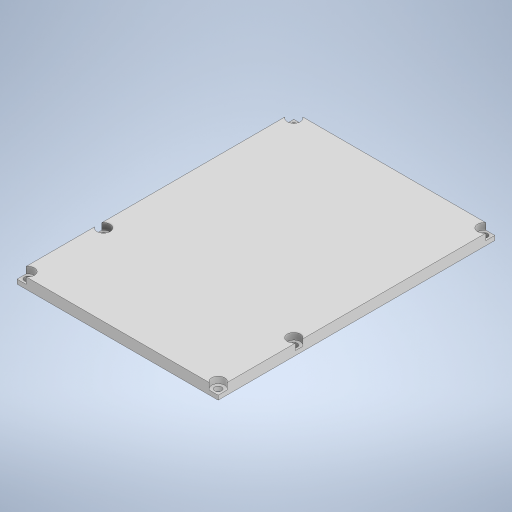
# Autodesk Inventor part: 싸피 뚜껑 원본
Saved by Autodesk Inventor 2023 (Build 270158000, 158)
## iProperties
Created: 2023-08-15
Part Number: 싸피 뚜껑 원본
Material: 일반
Document SubType Name: Sheet Metal
Designer: jin
Density: 1 g/cm^3
Sheet Metal Rule: 기본값_mm
Appearance: 기본값
Author: jin
## iProperties of the stored document 싸피 뚜껑_3D 인쇄.ipt
Created: 2023-08-16
Part Number: 싸피 뚜껑_3D 인쇄
Material: 일반
Document SubType Name: Modeling
Designer: jin
Density: 1 g/cm^3
Appearance: 기본값
Author: jin
Autodesk Inventor part; units mm, degrees
ref_plane "YZ Plane" through (0, 0, 0) normal (1, 0, 0) x (0, 1, 0)
ref_plane "XZ Plane" through (0, 0, 0) normal (0, 1, 0) x (-1, 0, 0)
ref_plane "XY Plane" through (0, 0, 0) normal (0, 0, 1) x (1, 0, 0)
sketch "스케치1" plane through (0, 0, 0) normal (0, 1, 0) x (-1, 0, 0)
  line L0 (0, 0) -> (93, 0)
  line L1 (93, 0) -> (93, -128)
  line L2 (93, -128) -> (0, -128)
  line L3 (0, -128) -> (0, 0)
  dimension "d0" = 93
  dimension "d1" = 128
  constraints: 8 end point, 2 parallel, 1 horizontal, 1 perpendicular
  measures "d0" distance of L1.end L2.end
  measures "d1" distance of L0.end L1.end
extrude "돌출1" add sketch "스케치1" along normal blind 5
sketch "스케치2" plane through (0, 5, 0) normal (0, 1, 0) x (1, 0, 0)
  line L0 (-93, 0) -> (0, 0) projected
  line L1 (0, 0) -> (0, 5)
  line L2 (0, 0) -> (0, 128) projected
  line L3 (0, 5) -> (0, 35)
  line L4 (0, 35) -> (0, 40)
  line L5 (0, 5) -> (-93, 5)
  line L6 (-93, 128) -> (-93, 0) projected
  line L7 (-93, 0) -> (-88, 0)
  line L8 (-88, 0) -> (-88, 5)
  line L9 (-88, 5) -> (-88, 35)
  line L10 (-88, 35) -> (0, 35)
  line L11 (-88, 35) -> (-93, 35)
  line L12 (-93, 35) -> (-93, 40)
  line L13 (-93, 40) -> (0, 40)
  line L14 (-88, 35) -> (-88, 40)
  line L15 (-88, 40) -> (-88, 128)
  line L16 (0, 128) -> (-93, 128) projected
  line L17 (-88, 128) -> (-88, 123)
  line L18 (-93, 123) -> (-88, 123)
  line L19 (-88, 123) -> (0, 123)
  line L20 (0, 128) -> (0, 125.5)
  line L21 (0, 125.5) -> (-2.5, 125.5)
  line L22 (-93, 128) -> (-93, 125.5)
  line L23 (-93, 125.5) -> (-90.5, 125.5)
  line L24 (-93, 40) -> (-93, 37.5)
  line L25 (-93, 37.5) -> (-90.5, 37.5)
  line L26 (0, 40) -> (0, 37.5)
  line L27 (0, 37.5) -> (-2.5, 37.5)
  line L28 (-93, 0) -> (-93, 2.5)
  line L29 (-93, 2.5) -> (-90.5, 2.5)
  line L30 (0, 0) -> (0, 2.5)
  line L31 (0, 5) -> (0, 2.5)
  line L32 (0, 2.5) -> (-2.5, 2.5)
  dimension "d4" = 5
  dimension "d5" = 30
  dimension "d6" = 5
  dimension "d7" = 5
  dimension "d8" = 30
  dimension "d9" = 5
  dimension "d10" = 5
  dimension "d11" = 2.5
  constraints: 58 end point, 20 point on line, 7 horizontal, 4 perpendicular, 2 midpoint, 1 collinear
  measures "d4" distance of L0.end L1.end
  measures "d5" distance of L1.end L3.end
  measures "d6" distance of L3.end L4.end
  measures "d7" distance of L0.start L7.end
  measures "d8" distance of L8.end L9.end
  measures "d9" distance of L11.end L12.end
  measures "d10" distance of L15.end L17.end
  measures "d11" distance of L20.end L21.end
hole "구멍1" at (-90.5, 5, -2.5) at (-2.5, 5, -2.5) at (-2.5, 5, -37.5) at (-90.5, 5, -37.5) at (-90.5, 5, -125.5) at (-2.5, 5, -125.5) direction (0, -1, 0) diameter 3.2 end through all counterbore diameter 6 counterbore depth 3
sketch "스케치4" plane through (0, 5, 0) normal (0, 1, 0) x (1, 0, 0)
  line L0 (-93.2831, -0.376) -> (-91.886, -0.376)
  line L1 (-91.886, -0.376) -> (-91.886, 1.0428)
  line L2 (-91.886, 1.0428) -> (-93.2831, 1.0428)
  line L3 (-93.2831, 1.0428) -> (-93.2831, -0.376)
  line L4 (-1.7168, -1.9392) -> (2.2785, -1.9392)
  line L5 (2.2785, -1.9392) -> (2.2785, 1.8635)
  line L6 (2.2785, 1.8635) -> (-1.7168, 1.8635)
  line L7 (-1.7168, 1.8635) -> (-1.7168, -1.9392)
  line L8 (-2.8454, 132.3005) -> (4.2676, 132.3005)
  line L9 (4.2676, 132.3005) -> (4.2676, 125.403)
  line L10 (4.2676, 125.403) -> (-2.8454, 125.403)
  line L11 (-2.8454, 125.403) -> (-2.8454, 132.3005)
  line L12 (-97.9012, 128.8517) -> (-90.3571, 128.8517)
  line L13 (-90.3571, 128.8517) -> (-90.3571, 125.403)
  line L14 (-90.3571, 125.403) -> (-97.9012, 125.403)
  line L15 (-97.9012, 125.403) -> (-97.9012, 128.8517)
  point P0 (0, 0)
  constraints: 32 end point, 8 parallel, 4 horizontal, 4 perpendicular, 1 point on line
extrude "돌출2" cut sketch "스케치4" against normal blind 3
equation "\"TransitionRadius\" = BendRadius"
equation "\"BendRadius\" = 0.5"
